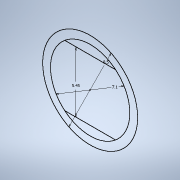
# Autodesk Inventor part: EncoderV2CAP
Saved by Autodesk Inventor 2022 (Build 260153070, 153G)
## iProperties
Created: 2022-01-31
Part Number: EncoderV2CAP
Material: Generic
Document SubType Name: Modeling
Designer: a laptop
Density: 1 g/cm^3
Appearance: Default
Author: a laptop
Autodesk Inventor part; units mm, degrees
ref_plane "YZ Plane" through (0, 0, 0) normal (1, 0, 0) x (0, 1, 0)
ref_plane "XZ Plane" through (0, 0, 0) normal (0, 1, 0) x (-1, 0, 0)
ref_plane "XY Plane" through (0, 0, 0) normal (0, 0, 1) x (1, 0, 0)
sketch "Sketch1" plane through (0, 0, 0) normal (0, 0, 1) x (1, 0, 0)
  circle A0 centre (0, 0) radius 3.55
  line L0 (-2.2753, 2.725) -> (2.2753, 2.725)
  line L1 (2.2753, -2.725) -> (-2.2753, -2.725)
  circle A1 centre (0, 0) radius 4.25
  dimension "d0" = 7.1
  dimension "d1" = 5.45
  dimension "d2" = 8.5
  constraints: 4 end point, 4 point on circle, 2 centre point, 2 coincident, 2 parallel, 1 horizontal
  measures "d0" diameter of A0
  measures "d1" distance between parallel lines of L1 L0
  measures "d2" diameter of A1
extrude "Extrusion1" add sketch "Sketch1" along normal blind 1.25 contours L0 A0 | A0 L1 | A1
sketch "Sketch4" plane through (0, 0, 1.25) normal (0, 0, 1) x (1, 0, 0)
  circle A0 centre (0, 0) radius 4.25 projected
  circle A1 centre (0, 0) radius 1
  dimension "d7" = 2
  constraints: 1 centre point, 1 coincident
  measures "d7" diameter of A1
extrude "Extrusion2" add sketch "Sketch4" along normal blind 1.25
fillet "Fillet1" radius 1 1 edges at (-4.25, 0, 2.5)
body "Solid1"
